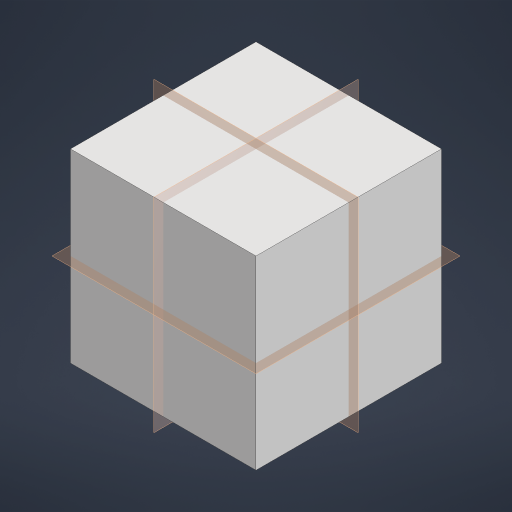
# Autodesk Inventor part: cube
Saved by Autodesk Inventor 2024 (Build 280153020, 153B)
## iProperties
Created: 2024-03-08
Part Number: cube
Material: Generic
Document SubType Name: Modeling
Designer: Oliver Read
Density: 1 g/cm^3
Appearance: Default
Author: Oliver Read
Autodesk Inventor part; units mm, degrees
(part 1 of 3)
sketch "Air Jet Form Tool" plane through (0, 0, 0) normal (0, 0, 1) x (1, 0, 0)
  line L0 (0.825, 4) -> (-0.795, 2.38)
  line L1 (-0.795, 2.38) -> (-2, 2.38)
  line L2 (-2, 2.38) -> (-2, 1.59)
  line L3 (-2, 1.59) -> (-4.8, 1.59)
  line L4 (-4.8, 1.59) -> (-4.8, 1.25)
  line L5 (-4.8, 1.25) -> (-8, 1.25)
  line L6 (-8, 1.25) -> (-9.25, 0)
  line L7 (0.825, 4) -> (0.825, 0)
  line L8 (0.825, 0) -> (-9.25, 0)
  point P0 (0, 0)
  point P1 (0, 0)
  point P2 (0, 3.175)
sketch "BS1 Centre Drill" plane through (0, 0, 0) normal (0, 0, 1) x (1, 0, 0)
  line L0 (0, 0) -> (1.5875, 0)
  line L1 (1.5875, 0) -> (0.595, -1.7191)
  line L2 (0.595, -1.7191) -> (0.595, -3.3455)
  line L3 (0.595, -3.3455) -> (0, -3.7031)
  line L4 (0, -3.7031) -> (0, 0)
sketch "BS2 Centre Drill" plane through (0, 0, 0) normal (0, 0, 1) x (1, 0, 0)
  line L0 (0, 0) -> (2.3812, 0)
  line L1 (2.3812, 0) -> (0.7937, -2.7496)
  line L2 (0.7937, -2.7496) -> (0.7938, -4.6349)
  line L3 (0.7938, -4.6349) -> (0, -5.1309)
  line L4 (0, -5.1309) -> (0, 0)
sketch "BS3 Centre Drill" plane through (0, 0, 0) normal (0, 0, 1) x (1, 0, 0)
  line L0 (0, 0) -> (3.175, 0)
  line L1 (3.175, 0) -> (1.1906, -3.437)
  line L2 (1.1906, -3.437) -> (1.1906, -6.6618)
  line L3 (1.1906, -6.6618) -> (0, -7.4058)
  line L4 (0, -7.4058) -> (0, 0)
sketch "BS4 Centre Drill" plane through (0, 0, 0) normal (0, 0, 1) x (1, 0, 0)
  line L0 (0, 0) -> (3.9688, 0)
  line L1 (3.9688, 0) -> (1.5875, -4.1244)
  line L2 (1.5875, -4.1244) -> (1.5875, -7.895)
  line L3 (1.5875, -7.895) -> (0, -8.8869)
  line L4 (0, -8.8869) -> (0, 0)
sketch "BS5 Centre Drill" plane through (0, 0, 0) normal (0, 0, 1) x (1, 0, 0)
  line L0 (0, 0) -> (5.5563, 0)
  line L1 (5.5563, 0) -> (2.3813, -5.4993)
  line L2 (2.3813, -5.4993) -> (2.3813, -11.155)
  line L3 (2.3813, -11.155) -> (0, -12.643)
  line L4 (0, -12.643) -> (0, 0)
sketch "CE - 5mm" plane through (0, 0, 0) normal (0, 0, 1) x (1, 0, 0)
  arc A0 (-0.75, 2.4875) -> (-0.75, -2.4875) centre (-1, 0) ccw
  arc A1 (-0.75, 1.7321) -> (-0.75, -1.7321) centre (-1, 0) ccw
  line L0 (-0.75, 1.7321) -> (-0.75, 2.4875)
  line L1 (-0.75, -2.4875) -> (-0.75, -1.7321)
  arc A2 (3.5, 2.4875) -> (3.5, -2.4875) centre (3.25, 0) ccw
  arc A3 (3.5, 1.7321) -> (1.5407, 0.375) centre (3.25, 0) ccw
  arc A4 (1.5407, -0.375) -> (3.5, -1.7321) centre (3.25, 0) ccw
  line L2 (3.5, 1.7321) -> (3.5, 2.4875)
  line L3 (3.5, -2.4875) -> (3.5, -1.7321)
  line L4 (3, -0.375) -> (3, 0.375)
  line L5 (1.5407, -0.375) -> (3, -0.375)
  line L6 (1.5407, 0.375) -> (3, 0.375)
  point P0 (0, 0)
sketch "UKCA - 5mm" plane through (0, 0, 0) normal (0, 0, 1) x (1, 0, 0)
  line L0 (1.0692, -0.2966) -> (0.6432, -0.2966) construction
  spline S0 degree 3 poles (1.0692, -0.2966) (0.6432, -0.2966) (0.2966, -0.6385) (0.2966, -1.0588) knots 1 1 1 1 2 2 2 2
  line L1 (0.6432, -0.2966) -> (0.2966, -0.6385) construction
  line L2 (0.2966, -0.6385) -> (0.2966, -1.0588) construction
  line L3 (0.2966, -1.0588) -> (0.2966, -2.5007)
  line L4 (0.2966, -2.5007) -> (0.7976, -2.5007)
  line L5 (-1.0692, 0.2966) -> (-1.7282, 0.2966)
  line L6 (0.7976, -1.9998) -> (1.9998, -1.9998)
  line L7 (1.9998, -1.9998) -> (1.9998, -2.5007)
  line L8 (1.9998, -2.5007) -> (2.5007, -2.5007)
  line L9 (2.5007, -2.5007) -> (2.5007, -1.0588)
  spline S1 degree 3 poles (2.5007, -1.0588) (2.5007, -0.6385) (2.1542, -0.2966) (1.7282, -0.2966) knots 9 9 9 9 10 10 10 10
  line L10 (2.5007, -1.0588) -> (2.5007, -0.6385) construction
  line L11 (2.5007, -0.6385) -> (2.1542, -0.2966) construction
  line L12 (2.1542, -0.2966) -> (1.7282, -0.2966) construction
  line L13 (0.7976, -2.5007) -> (0.7976, -1.9998)
  spline S2 degree 3 poles (0.7976, -1.0655) (0.7976, -0.9178) (0.9224, -0.7975) (1.0759, -0.7975) knots 1 1 1 1 2 2 2 2
  line L14 (0.7976, -1.0655) -> (0.7976, -0.9178) construction
  line L15 (0.7976, -0.9178) -> (0.9224, -0.7975) construction
  line L16 (0.9224, -0.7975) -> (1.0759, -0.7975) construction
  line L17 (1.0759, -0.7975) -> (1.7215, -0.7975)
  spline S3 degree 3 poles (1.7215, -0.7975) (1.8749, -0.7975) (1.9998, -0.9178) (1.9998, -1.0655) knots 3 3 3 3 4 4 4 4
  line L18 (1.7215, -0.7975) -> (1.8749, -0.7975) construction
  line L19 (1.8749, -0.7975) -> (1.9998, -0.9178) construction
  line L20 (1.9998, -0.9178) -> (1.9998, -1.0655) construction
  line L21 (1.9998, -1.0655) -> (1.9998, -1.4988)
  line L22 (1.9998, -1.4988) -> (0.7976, -1.4988)
  line L23 (0.7976, -1.4988) -> (0.7976, -1.0655)
  line L24 (-0.4795, 2.5007) -> (-0.4604, 2.5007)
  spline S4 degree 3 poles (-1.7282, 0.2966) (-2.1542, 0.2966) (-2.5007, 0.6386) (-2.5007, 1.0588) knots 1 1 1 1 2 2 2 2
  line L25 (-1.7282, 0.2966) -> (-2.1542, 0.2966) construction
  line L26 (-2.1542, 0.2966) -> (-2.5007, 0.6386) construction
  line L27 (-2.5007, 0.6386) -> (-2.5007, 1.0588) construction
  line L28 (-2.5007, 1.0588) -> (-2.5007, 2.5007)
  line L29 (-2.5007, 2.5007) -> (-1.9998, 2.5007)
  line L30 (-1.9998, 2.5007) -> (-1.9998, 1.0656)
  spline S5 degree 3 poles (-1.9998, 1.0656) (-1.9998, 0.9178) (-1.8749, 0.7976) (-1.7215, 0.7976) knots 5 5 5 5 6 6 6 6
  line L31 (-1.9998, 1.0656) -> (-1.9998, 0.9178) construction
  line L32 (-1.9998, 0.9178) -> (-1.8749, 0.7976) construction
  line L33 (-1.8749, 0.7976) -> (-1.7215, 0.7976) construction
  line L34 (-1.7215, 0.7976) -> (-1.0759, 0.7976)
  spline S6 degree 3 poles (-1.0759, 0.7976) (-0.9224, 0.7976) (-0.7976, 0.9178) (-0.7976, 1.0656) knots 7 7 7 7 8 8 8 8
  line L35 (-1.0759, 0.7976) -> (-0.9224, 0.7976) construction
  line L36 (-0.9224, 0.7976) -> (-0.7976, 0.9178) construction
  line L37 (-0.7976, 0.9178) -> (-0.7976, 1.0656) construction
  line L38 (-0.7976, 1.0656) -> (-0.7976, 2.5007)
  line L39 (-0.7976, 2.5007) -> (-0.2966, 2.5007)
  line L40 (-0.2966, 2.5007) -> (-0.2966, 1.0588)
  spline S7 degree 3 poles (-0.2966, 1.0588) (-0.2966, 0.6386) (-0.6432, 0.2966) (-1.0692, 0.2966) knots 11 11 11 11 12 12 12 12
  line L41 (-0.2966, 1.0588) -> (-0.2966, 0.6386) construction
  line L42 (-0.2966, 0.6386) -> (-0.6432, 0.2966) construction
  line L43 (-0.6432, 0.2966) -> (-1.0692, 0.2966) construction
  line L44 (2.5053, 2.5007) -> (1.8575, 2.5007)
  line L45 (1.8575, 2.5007) -> (0.7976, 1.6666)
  line L46 (0.7976, 1.6666) -> (0.7976, 2.5007)
  line L47 (0.7976, 2.5007) -> (0.2966, 2.5007)
  line L48 (0.2966, 2.5007) -> (0.2966, 0.2966)
  line L49 (0.2966, 0.2966) -> (0.7976, 0.2966)
  line L50 (0.7976, 0.2966) -> (0.7976, 1.1363)
  line L51 (0.7976, 1.1363) -> (1.8575, 0.2966)
  line L52 (1.8575, 0.2966) -> (2.5025, 0.2966)
  line L53 (2.5025, 0.2966) -> (1.1082, 1.4012)
  line L54 (1.1082, 1.4012) -> (2.5053, 2.5007)
  line L55 (-0.2966, -2.5007) -> (-1.7385, -2.5007)
  spline S8 degree 3 poles (-1.7385, -2.5007) (-2.1588, -2.5007) (-2.5007, -2.1474) (-2.5007, -1.7215) knots 1 1 1 1 2 2 2 2
  line L56 (-1.7385, -2.5007) -> (-2.1588, -2.5007) construction
  line L57 (-2.1588, -2.5007) -> (-2.5007, -2.1474) construction
  line L58 (-2.5007, -2.1474) -> (-2.5007, -1.7215) construction
  line L59 (-2.5007, -1.7215) -> (-2.5007, -1.0759)
  spline S9 degree 3 poles (-2.5007, -1.0759) (-2.5007, -0.6499) (-2.1588, -0.2966) (-1.7385, -0.2966) knots 3 3 3 3 4 4 4 4
  line L60 (-2.5007, -1.0759) -> (-2.5007, -0.6499) construction
  line L61 (-2.5007, -0.6499) -> (-2.1588, -0.2966) construction
  line L62 (-2.1588, -0.2966) -> (-1.7385, -0.2966) construction
  line L63 (-1.7385, -0.2966) -> (-0.2966, -0.2966)
  line L64 (-0.2966, -0.2966) -> (-0.2966, -0.7976)
  line L65 (-0.2966, -0.7976) -> (-1.7318, -0.7976)
  spline S10 degree 3 poles (-1.7318, -0.7976) (-1.8796, -0.7976) (-1.9998, -0.9224) (-1.9998, -1.0759) knots 7 7 7 7 8 8 8 8
  line L66 (-1.7318, -0.7976) -> (-1.8796, -0.7976) construction
  line L67 (-1.8796, -0.7976) -> (-1.9998, -0.9224) construction
  line L68 (-1.9998, -0.9224) -> (-1.9998, -1.0759) construction
  line L69 (-1.9998, -1.0759) -> (-1.9998, -1.7215)
  spline S11 degree 3 poles (-1.9998, -1.7215) (-1.9998, -1.8749) (-1.8796, -1.9998) (-1.7318, -1.9998) knots 9 9 9 9 10 10 10 10
  line L70 (-1.9998, -1.7215) -> (-1.9998, -1.8749) construction
  line L71 (-1.9998, -1.8749) -> (-1.8796, -1.9998) construction
  line L72 (-1.8796, -1.9998) -> (-1.7318, -1.9998) construction
  line L73 (-1.7318, -1.9998) -> (-0.2966, -1.9998)
  line L74 (-0.2966, -1.9998) -> (-0.2966, -2.5007)
  line L75 (1.7282, -0.2966) -> (1.0692, -0.2966)
  point P0 (0, 0)
sketch "WEEE - 5mm" plane through (0, 0, 0) normal (0, 0, 1) x (1, 0, 0)
  line L0 (1.7158, 2.5006) -> (1.7167, 2.5006)
  line L1 (-1.4262, -1.7883) -> (1.4264, -1.7883)
  line L2 (1.4264, -1.7883) -> (1.4264, -2.501)
  line L3 (1.4264, -2.501) -> (-1.4262, -2.501)
  circle A0 centre (0.5816, -0.4361) radius 0.0929
  arc A1 (0.5682, -0.1516) -> (0.3027, -0.4944) centre (0.5816, -0.4361) ccw
  arc A2 (0.3256, -0.5612) -> (0.8613, -0.382) centre (0.5816, -0.4361) ccw
  line L4 (0.3027, -0.4944) -> (-0.5023, -0.4944)
  line L5 (-0.5023, -0.4944) -> (-0.5485, 0.0433)
  line L6 (-0.5569, 0.1401) -> (-0.653, 1.2575)
  line L7 (-0.6619, 1.3613) -> (-0.6998, 1.8018)
  line L8 (0.3256, -0.5612) -> (-0.3706, -0.5612)
  line L9 (-0.3706, -0.5612) -> (-0.3706, -0.7192)
  line L10 (-0.3706, -0.7192) -> (-0.5415, -0.7192)
  line L11 (-0.5415, -0.7192) -> (-0.5415, -0.5602)
  arc A3 (-0.5811, -0.5036) -> (-0.5415, -0.5602) centre (-0.5214, -0.5041) ccw
  line L12 (-0.5811, -0.5041) -> (-0.6215, -0.0326)
  line L13 (-0.6299, 0.0642) -> (-0.7405, 1.3522)
  line L14 (-0.7494, 1.4557) -> (-0.7791, 1.8015)
  line L15 (-0.7791, 1.8015) -> (-0.9112, 1.8015)
  line L16 (-0.9112, 1.8015) -> (-0.9112, 1.8938)
  line L17 (-0.9112, 1.8938) -> (-0.7925, 1.8938)
  line L18 (-0.7139, 1.8938) -> (-0.6074, 1.8938)
  line L19 (-0.436, 1.8938) -> (0.7146, 1.8938)
  line L20 (-0.6998, 1.8018) -> (0.7133, 1.8018)
  line L21 (0.7133, 1.8018) -> (0.6996, 1.6165)
  line L22 (0.6751, 1.287) -> (0.5808, 0.0185)
  line L23 (0.5741, -0.0711) -> (0.5682, -0.1516)
  line L24 (0.7799, 1.8115) -> (0.7663, 1.6162)
  line L25 (0.7434, 1.287) -> (0.65, -0.0563)
  circle A4 centre (0.5816, -0.4361) radius 0.1555
  line L26 (-0.6074, 1.8938) -> (-0.6074, 2.0043)
  line L27 (-0.6074, 2.0851) -> (-0.6074, 2.1583)
  line L28 (-0.6074, 2.1583) -> (-0.436, 2.1583)
  line L29 (-0.436, 2.1583) -> (-0.436, 2.1445)
  line L30 (-0.436, 2.0657) -> (-0.436, 1.8938)
  arc A5 (-0.688, 1.9531) -> (-0.7139, 1.8938) centre (-0.6372, 1.8957) ccw
  arc A6 (-0.6074, 2.0043) -> (-0.688, 1.9531) centre (-0.3127, 1.4513) ccw
  arc A7 (-0.1585, 2.0919) -> (-0.436, 2.0657) centre (-0.1257, 0.2588) ccw
  arc A8 (-0.1585, 2.1706) -> (-0.436, 2.1445) centre (-0.1257, 0.3376) ccw
  line L31 (-0.1585, 2.2104) -> (-0.1585, 2.1706)
  line L32 (-0.1585, 2.0919) -> (-0.1585, 1.9995)
  line L33 (-0.1585, 1.9995) -> (0.2905, 1.9995)
  line L34 (0.2905, 1.9995) -> (0.2905, 2.0905)
  line L35 (0.2905, 2.1631) -> (0.2905, 2.2104)
  line L36 (0.2905, 2.2104) -> (-0.1585, 2.2104)
  line L37 (-0.0924, 2.1315) -> (-0.0924, 2.0789)
  line L38 (-0.0924, 2.0789) -> (0.2244, 2.0789)
  line L39 (0.2244, 2.0789) -> (0.2244, 2.1315)
  line L40 (0.2244, 2.1315) -> (-0.0924, 2.1315)
  arc A9 (-0.7663, 1.9743) -> (-0.7925, 1.8938) centre (-0.6917, 1.9054) ccw
  arc A10 (-0.6074, 2.0851) -> (-0.7663, 1.9743) centre (-0.2997, 1.4745) ccw
  arc A11 (0.7799, 1.8115) -> (0.7427, 1.9727) centre (0.8536, 1.9134) ccw
  arc A12 (0.6431, 1.9765) -> (0.4637, 2.0618) centre (0.3184, 1.5254) ccw
  arc A13 (0.7146, 1.8938) -> (0.6431, 1.9765) centre (0.5326, 1.8085) ccw
  arc A14 (0.617, 2.0738) -> (0.2905, 2.1631) centre (0.2581, 1.4034) ccw
  arc A15 (0.7427, 1.9727) -> (0.617, 2.0738) centre (0.3672, 1.6344) ccw
  arc A16 (0.4637, 2.0618) -> (0.2905, 2.0905) centre (0.1785, 0.8757) ccw
  line L41 (0.6603, 1.287) -> (0.6751, 1.287)
  line L42 (0.7434, 1.287) -> (0.9769, 1.287)
  line L43 (0.9769, 1.287) -> (0.9769, 1.6165)
  line L44 (0.6603, 1.6165) -> (0.6996, 1.6165)
  line L45 (0.7663, 1.6162) -> (0.8644, 1.6162)
  line L46 (0.9519, 1.6165) -> (0.9769, 1.6165)
  line L47 (0.6603, 1.6165) -> (0.6603, 1.4045)
  line L48 (0.6603, 1.3003) -> (0.6603, 1.287)
  line L49 (0.7522, 1.4058) -> (0.7522, 1.3659)
  line L50 (0.7522, 1.3659) -> (0.9112, 1.3659)
  line L51 (0.9112, 1.3659) -> (0.9112, 1.551)
  line L52 (0.9112, 1.551) -> (0.8981, 1.551)
  line L53 (0.7522, 1.4058) -> (0.8981, 1.551)
  line L54 (0.6603, 1.3003) -> (0.0153, 0.6296)
  line L55 (-1.4262, -2.501) -> (-1.4262, -1.7883)
  line L56 (-0.6215, -0.0326) -> (-1.6049, -1.0552)
  line L57 (-1.6049, -1.0552) -> (-1.657, -1.0028)
  line L58 (-1.657, -1.0028) -> (-0.6299, 0.0642)
  line L59 (-0.5569, 0.1401) -> (-0.0792, 0.6363)
  line L60 (-0.0342, 0.683) -> (0.3565, 1.0889)
  line L61 (0.4223, 1.1572) -> (0.6603, 1.4045)
  line L62 (0.8644, 1.6162) -> (1.7158, 2.5006)
  line L63 (1.7167, 2.5006) -> (1.7167, 2.4087)
  line L64 (1.7167, 2.4087) -> (0.9519, 1.6165)
  line L65 (0.4223, 1.1572) -> (0.4223, 1.2734)
  line L66 (0.4223, 1.2734) -> (-0.1717, 1.2734)
  line L67 (-0.0298, 0.5827) -> (-0.5485, 0.0433)
  line L68 (-0.1717, 1.0889) -> (0.3565, 1.0889)
  line L69 (-1.7167, 2.501) -> (-1.7167, 2.4092)
  line L70 (-1.7167, 2.4092) -> (-0.7405, 1.3522)
  line L71 (-0.653, 1.2575) -> (-0.0792, 0.6363)
  line L72 (-0.0298, 0.5827) -> (0.5741, -0.0711)
  line L73 (0.8613, -0.382) -> (1.4837, -1.0559)
  line L74 (1.4837, -1.0559) -> (1.533, -1.0104)
  line L75 (1.533, -1.0104) -> (0.65, -0.0563)
  line L76 (0.5808, 0.0185) -> (0.0153, 0.6296)
  line L77 (-0.0342, 0.683) -> (-0.6619, 1.3613)
  line L78 (-0.7494, 1.4557) -> (-1.7167, 2.501)
  line L79 (-0.1717, 1.2734) -> (-0.1717, 1.0889)
  point P0 (0, 0)
sketch "TELEC - 5mm" plane through (0, 0, 0) normal (0, 0, 1) x (1, 0, 0)
  arc A0 (0.4326, 0.6165) -> (0.3669, -0.8333) centre (-1.9901, 0) ccw
  arc A1 (0.0002, 0.8562) -> (-4.059, 0.6437) centre (-1.9901, 0) ccw
  line L0 (-3.3235, -0.8333) -> (-0.6568, -0.8333)
  line L1 (-0.6568, -0.8333) -> (-0.6568, -1.25)
  line L2 (-2.2401, -1.9167) -> (-1.7401, -1.9167)
  line L3 (-1.7401, -1.25) -> (-1.7401, -1.9167)
  line L4 (-1.7401, -1.25) -> (-0.6568, -1.25)
  line L5 (-2.2401, -1.25) -> (-2.2401, -1.9167)
  line L6 (-2.2401, -1.25) -> (-3.3235, -1.25)
  line L7 (-3.3235, -0.8333) -> (-3.3235, -1.25)
  line L8 (-3.3235, -0.5833) -> (-0.6568, -0.5833)
  line L9 (-0.6568, -0.5833) -> (-0.6568, -0.1667)
  line L10 (-3.3235, -0.5833) -> (-3.3235, -0.1667)
  line L11 (-3.3235, -0.1667) -> (-0.6568, -0.1667)
  line L12 (-2.1568, 0) -> (0.4326, 0.6165)
  line L13 (-4.1384, 0.2822) -> (-2.1568, 0.754)
  line L14 (-2.1568, 0) -> (-2.1568, 0.754)
  line L15 (-1.8235, 0.422) -> (0.0002, 0.8562)
  line L16 (-1.8235, 0.422) -> (-1.8235, 1.176)
  line L17 (-4.059, 0.6437) -> (-1.8235, 1.176)
  arc A2 (-4.1384, 0.2822) -> (0.0099, -0.8333) centre (-1.9901, 0) ccw
  line L18 (0.0099, -0.8333) -> (0.3669, -0.8333)
  line L19 (1.9123, 0.6959) -> (4.4042, 0.6959)
  line L20 (4.4042, 0.6959) -> (4.4042, -2.0609)
  line L21 (4.4042, -2.0609) -> (1.9123, -2.0609)
  line L22 (1.9123, -2.0609) -> (1.9123, 0.6959)
  line L23 (1.829, 0.7793) -> (4.4876, 0.7793)
  line L24 (4.4876, 0.7793) -> (4.4876, -2.1442)
  line L25 (4.4876, -2.1442) -> (1.829, -2.1442)
  line L26 (1.829, -2.1442) -> (1.829, 0.7793)
  line L27 (2.2996, 0.346) -> (2.2996, -1.7374)
  line L28 (2.2996, -1.7374) -> (2.7162, -1.7374)
  line L29 (2.7162, -1.7374) -> (2.7162, -0.8624)
  line L30 (2.7162, -0.8624) -> (2.9324, -0.8624)
  line L31 (3.6746, -1.7374) -> (4.1746, -1.7374)
  arc A3 (4.1746, -1.7374) -> (3.4751, -0.8264) centre (1.4812, -3.0813) ccw
  arc A4 (3.6746, -1.7374) -> (3.0775, -0.9212) centre (0.9812, -3.0813) ccw
  arc A5 (3.0775, -0.9212) -> (2.9324, -0.8624) centre (2.9324, -1.0707) ccw
  line L32 (2.7018, 0.015) -> (2.7018, -0.5017)
  arc A6 (3.3268, -0.5017) -> (3.3268, 0.015) centre (3.3268, -0.2433) ccw
  line L33 (2.7018, 0.015) -> (3.3268, 0.015)
  line L34 (3.3268, -0.5017) -> (2.7018, -0.5017)
  line L35 (2.2996, 0.346) -> (3.3895, 0.346)
  arc A7 (3.4751, -0.8264) -> (3.3895, 0.346) centre (3.3895, -0.2433) ccw
  point P0 (0, 0)
sketch "KCC - 5mm" plane through (0, 0, 0) normal (0, 0, 1) x (1, 0, 0)
  arc A0 (0.975, 0.9255) -> (0.975, -0.9255) centre (1.2235, 0) ccw
  arc A1 (1.0408, 0.9341) -> (0.975, 0.9255) centre (1.0408, 0.6805) ccw
  line L0 (1.0408, 0.9341) -> (1.6027, 0.9341)
  line L1 (1.6027, 0.9341) -> (1.6027, 0.6316)
  line L2 (1.6027, 0.6316) -> (1.1105, 0.6316)
  arc A2 (1.1105, 0.6316) -> (1.0378, 0.621) centre (1.1105, 0.378) ccw
  arc A3 (1.0378, 0.621) -> (1.0378, -0.621) centre (1.2235, 0) ccw
  arc A4 (1.0378, -0.621) -> (1.1105, -0.6316) centre (1.1105, -0.378) ccw
  line L3 (1.1105, -0.6316) -> (1.6027, -0.6316)
  line L4 (1.6027, -0.6316) -> (1.6027, -1.7334)
  line L5 (1.6027, -1.7334) -> (1.0569, -1.7334)
  arc A5 (1.0285, -1.7319) -> (1.0569, -1.7334) centre (1.0569, -1.4798) ccw
  arc A6 (1.0285, 1.7319) -> (1.0285, -1.7319) centre (1.2235, 0) ccw
  arc A7 (1.0569, 1.7334) -> (1.0285, 1.7319) centre (1.0569, 1.4798) ccw
  line L6 (1.0569, 1.7334) -> (1.2987, 1.7334)
  line L7 (1.2987, 1.7334) -> (1.2987, 2.179)
  line L8 (1.2987, 2.179) -> (1.0597, 2.179)
  arc A8 (1.0597, 2.179) -> (1.0382, 2.1781) centre (1.0597, 1.9253) ccw
  arc A9 (1.0382, 2.1781) -> (-0.8208, 0.774) centre (1.2235, 0) ccw
  line L9 (-0.8208, 0.774) -> (-0.8208, 2.1281)
  line L10 (-0.8208, 2.1281) -> (-1.2971, 2.1281)
  line L11 (-1.2971, 2.1281) -> (-1.2971, -2.1932)
  line L12 (-1.2971, -2.1932) -> (-0.8208, -2.1932)
  line L13 (-0.8208, -2.1932) -> (-0.8208, -0.774)
  arc A10 (-0.8208, -0.774) -> (1.0382, -2.1781) centre (1.2235, 0) ccw
  arc A11 (1.0382, -2.1781) -> (1.0597, -2.179) centre (1.0597, -1.9253) ccw
  line L14 (1.0597, -2.179) -> (1.6027, -2.179)
  line L15 (1.6027, -2.179) -> (1.6027, -2.5)
  line L16 (1.6027, -2.5) -> (0.9791, -2.5)
  arc A12 (0.9517, -2.4985) -> (0.9791, -2.5) centre (0.9791, -2.2463) ccw
  arc A13 (-0.5344, -1.7962) -> (0.9517, -2.4985) centre (1.2235, 0) ccw
  line L17 (-0.5344, -1.7962) -> (-0.5344, -2.5)
  line L18 (-0.5344, -2.5) -> (-1.6027, -2.5)
  line L19 (-1.6027, -2.5) -> (-1.6027, 2.5)
  line L20 (-1.6027, 2.5) -> (-0.5344, 2.5)
  line L21 (-0.5344, 2.5) -> (-0.5344, 1.7962)
  arc A14 (0.9517, 2.4985) -> (-0.5344, 1.7962) centre (1.2235, 0) ccw
  arc A15 (0.9791, 2.5) -> (0.9517, 2.4985) centre (0.9791, 2.2463) ccw
  line L22 (0.9791, 2.5) -> (1.6027, 2.5)
  line L23 (1.6027, 2.5) -> (1.6027, 1.4133)
  line L24 (1.6027, 1.4133) -> (1.0559, 1.4133)
  arc A16 (1.0559, 1.4133) -> (1.0196, 1.4107) centre (1.0559, 1.1596) ccw
  arc A17 (1.0196, 1.4107) -> (1.0196, -1.4107) centre (1.2235, 0) ccw
  arc A18 (1.0196, -1.4107) -> (1.0559, -1.4133) centre (1.0559, -1.1596) ccw
  line L25 (1.0559, -1.4133) -> (1.2987, -1.4133)
  line L26 (1.2987, -1.4133) -> (1.2987, -0.9341)
  line L27 (1.2987, -0.9341) -> (1.0408, -0.9341)
  arc A19 (0.975, -0.9255) -> (1.0408, -0.9341) centre (1.0408, -0.6805) ccw
  point P0 (0, 0)
sketch "Bowers Logo 1" plane through (0, 0, 0) normal (0, 0, 1) x (1, 0, 0)
  line L0 (0.7957, 3.45) -> (1.2479, 4.8418)
  line L1 (0.7957, 3.45) -> (1.2479, 4.8418)
  line L2 (-1.0969, 3.45) -> (0.7957, 3.45)
  line L3 (-1.0969, 3.45) -> (0.7957, 3.45)
  line L4 (-3.1926, -3) -> (-1.0969, 3.45)
  line L5 (-3.1926, -3) -> (-1.0969, 3.45)
  line L6 (-1.3, -3) -> (-3.1926, -3)
  line L7 (-1.3, -3) -> (-3.1926, -3)
  line L8 (-1.8363, -4.6506) -> (-1.3, -3)
  line L9 (-1.8363, -4.6506) -> (-1.3, -3)
  arc A0 (1.2479, 4.8418) -> (-1.8363, -4.6506) centre (0, 0) ccw
  line L10 (-1.8363, -4.6506) -> (-1.3, -3)
  line L11 (-1.3, -3) -> (-3.1926, -3)
  line L12 (-3.1926, -3) -> (-1.0969, 3.45)
  line L13 (-1.0969, 3.45) -> (0.7957, 3.45)
  line L14 (0.7957, 3.45) -> (1.2479, 4.8418)
  arc A1 (1.2479, 4.8418) -> (-1.8363, -4.6506) centre (0, 0) ccw
  line L15 (0.7957, 3.45) -> (1.2479, 4.8418)
  line L16 (-1.0969, 3.45) -> (0.7957, 3.45)
  line L17 (-3.1926, -3) -> (-1.0969, 3.45)
  line L18 (-1.3, -3) -> (-3.1926, -3)
  line L19 (-1.8363, -4.6506) -> (-1.3, -3)
  line L20 (2.1463, 4.5159) -> (1.8, 3.45)
  line L21 (2.1463, 4.5159) -> (1.8, 3.45)
  line L22 (-0.34, -3) -> (-0.9596, -4.907)
  line L23 (-0.34, -3) -> (-0.9596, -4.907)
  line L24 (1.76, -3) -> (-0.34, -3)
  line L25 (1.76, -3) -> (-0.34, -3)
  arc A2 (1.76, -3) -> (2.5364, 0.8349) centre (1.4, -0.9311) ccw
  line L26 (1.76, -3) -> (-0.34, -3)
  line L27 (-0.34, -3) -> (-0.9596, -4.907)
  arc A3 (-0.9596, -4.907) -> (2.1463, 4.5159) centre (0, 0) ccw
  line L28 (2.1463, 4.5159) -> (1.8, 3.45)
  arc A4 (2.5364, 0.8349) -> (1.8, 3.45) centre (1.5559, 1.97) ccw
  arc A5 (1.76, -3) -> (2.5364, 0.8349) centre (1.4, -0.9311) ccw
  arc A6 (2.5364, 0.8349) -> (1.8, 3.45) centre (1.5559, 1.97) ccw
  line L29 (2.1463, 4.5159) -> (1.8, 3.45)
  arc A7 (-0.9596, -4.907) -> (2.1463, 4.5159) centre (0, 0) ccw
  line L30 (-0.34, -3) -> (-0.9596, -4.907)
  line L31 (1.76, -3) -> (-0.34, -3)
  line L32 (-0.34, -3) -> (1.8, 3.45)
  line L33 (-0.34, -3) -> (1.8, 3.45)
  line L34 (-1.3, -3) -> (-0.34, -3)
  line L35 (-1.3, -3) -> (-0.34, -3)
  line L36 (0.7957, 3.45) -> (-1.3, -3)
  line L37 (0.7957, 3.45) -> (-1.3, -3)
  line L38 (1.8, 3.45) -> (0.7957, 3.45)
  line L39 (1.8, 3.45) -> (0.7957, 3.45)
  line L40 (1.8, 3.45) -> (0.7957, 3.45)
  line L41 (0.7957, 3.45) -> (-1.3, -3)
  line L42 (-1.3, -3) -> (-0.34, -3)
  line L43 (-0.34, -3) -> (1.8, 3.45)
  line L44 (1.8, 3.45) -> (0.7957, 3.45)
  line L45 (-0.34, -3) -> (1.8, 3.45)
  line L46 (-1.3, -3) -> (-0.34, -3)
  line L47 (0.7957, 3.45) -> (-1.3, -3)
  point P0 (0, 0)
sketch "Bowers Logo 2" plane through (0, 0, 0) normal (0, 0, 1) x (1, 0, 0)
  arc A0 (-15.0251, -2.8294) -> (-14.9267, -1.9003) centre (-15.0392, -2.3581) ccw
  line L0 (-15.0251, -2.8294) -> (-15.6547, -2.8294)
  line L1 (-14.9267, -1.9003) -> (-15.4912, -1.9003)
  line L2 (10.3315, -2.1386) -> (10.4158, -2.1472)
  line L3 (10.4158, -2.1472) -> (10.3315, -2.1386)
  line L4 (10.4158, -2.1472) -> (10.4958, -2.1638)
  line L5 (10.4958, -2.1638) -> (10.4158, -2.1472)
  line L6 (10.4958, -2.1638) -> (10.573, -2.189)
  line L7 (10.573, -2.189) -> (10.4958, -2.1638)
  line L8 (10.573, -2.189) -> (10.6458, -2.2222)
  line L9 (10.6458, -2.2222) -> (10.573, -2.189)
  line L10 (10.6458, -2.2222) -> (10.715, -2.2647)
  line L11 (10.715, -2.2647) -> (10.6458, -2.2222)
  line L12 (10.715, -2.2647) -> (10.7806, -2.3152)
  line L13 (10.7806, -2.3152) -> (10.715, -2.2647)
  line L14 (10.7806, -2.3152) -> (10.8419, -2.3743)
  line L15 (10.8419, -2.3743) -> (10.7806, -2.3152)
  line L16 (10.8419, -2.3743) -> (10.8578, -2.3909)
  line L17 (10.8578, -2.3909) -> (10.8419, -2.3743)
  line L18 (10.8578, -2.3909) -> (10.9061, -2.4522)
  line L19 (10.9061, -2.4522) -> (10.8578, -2.3909)
  line L20 (10.9061, -2.4522) -> (10.9479, -2.5178)
  line L21 (10.9479, -2.5178) -> (10.9061, -2.4522)
  line L22 (10.9479, -2.5178) -> (10.9832, -2.5877)
  line L23 (10.9832, -2.5877) -> (10.9479, -2.5178)
  line L24 (10.9832, -2.5877) -> (11.0128, -2.6627)
  line L25 (11.0128, -2.6627) -> (10.9832, -2.5877)
  line L26 (11.0128, -2.6627) -> (11.0351, -2.742)
  line L27 (11.0351, -2.742) -> (11.0128, -2.6627)
  line L28 (11.0351, -2.742) -> (11.051, -2.8264)
  line L29 (11.051, -2.8264) -> (11.0351, -2.742)
  line L30 (11.051, -2.8264) -> (11.0611, -2.9151)
  line L31 (11.0611, -2.9151) -> (11.051, -2.8264)
  line L32 (11.0611, -2.9151) -> (11.064, -3.0088)
  line L33 (11.064, -3.0088) -> (11.0611, -2.9151)
  line L34 (11.064, -3.0088) -> (11.0618, -3.0902)
  line L35 (11.0618, -3.0902) -> (11.064, -3.0088)
  line L36 (11.0618, -3.0902) -> (11.0546, -3.1732)
  line L37 (11.0546, -3.1732) -> (11.0618, -3.0902)
  line L38 (11.0546, -3.1732) -> (11.0431, -3.2561)
  line L39 (11.0431, -3.2561) -> (11.0546, -3.1732)
  line L40 (11.0431, -3.2561) -> (11.0272, -3.3397)
  line L41 (11.0272, -3.3397) -> (11.0431, -3.2561)
  line L42 (11.0272, -3.3397) -> (11.0063, -3.4233)
  line L43 (11.0063, -3.4233) -> (11.0272, -3.3397)
  line L44 (11.0063, -3.4233) -> (10.9803, -3.5077)
  line L45 (10.9803, -3.5077) -> (11.0063, -3.4233)
  line L46 (10.9803, -3.5077) -> (10.9565, -3.5747)
  line L47 (10.9565, -3.5747) -> (10.9803, -3.5077)
  line L48 (10.9565, -3.5747) -> (10.9219, -3.6562)
  line L49 (10.9219, -3.6562) -> (10.9565, -3.5747)
  line L50 (10.9219, -3.6562) -> (10.8844, -3.7333)
  line L51 (10.8844, -3.7333) -> (10.9219, -3.6562)
  line L52 (10.8844, -3.7333) -> (10.8433, -3.8054)
  line L53 (10.8433, -3.8054) -> (10.8844, -3.7333)
  line L54 (10.8433, -3.8054) -> (10.7979, -3.8725)
  line L55 (10.7979, -3.8725) -> (10.8433, -3.8054)
  line L56 (10.7979, -3.8725) -> (10.7496, -3.9352)
  line L57 (10.7496, -3.9352) -> (10.7979, -3.8725)
  line L58 (10.7496, -3.9352) -> (10.7431, -3.9424)
  line L59 (10.7431, -3.9424) -> (10.7496, -3.9352)
  line L60 (10.7431, -3.9424) -> (10.684, -4.0073)
  line L61 (10.684, -4.0073) -> (10.7431, -3.9424)
  line L62 (10.684, -4.0073) -> (10.6213, -4.0657)
  line L63 (10.6213, -4.0657) -> (10.684, -4.0073)
  line L64 (10.6213, -4.0657) -> (10.5564, -4.1183)
  line L65 (10.5564, -4.1183) -> (10.6213, -4.0657)
  line L66 (10.5564, -4.1183) -> (10.4879, -4.1652)
  line L67 (10.4879, -4.1652) -> (10.5564, -4.1183)
  line L68 (10.4879, -4.1652) -> (10.4165, -4.2063)
  line L69 (10.4165, -4.2063) -> (10.4879, -4.1652)
  line L70 (10.4165, -4.2063) -> (10.3524, -4.2366)
  line L71 (10.3524, -4.2366) -> (10.4165, -4.2063)
  line L72 (10.3524, -4.2366) -> (10.2731, -4.2661)
  line L73 (10.2731, -4.2661) -> (10.3524, -4.2366)
  line L74 (10.2731, -4.2661) -> (10.1923, -4.287)
  line L75 (10.1923, -4.287) -> (10.2731, -4.2661)
  line L76 (10.1923, -4.287) -> (10.1101, -4.3)
  line L77 (10.1101, -4.3) -> (10.1923, -4.287)
  line L78 (10.1101, -4.3) -> (10.0258, -4.3043)
  line L79 (10.0258, -4.3043) -> (10.1101, -4.3)
  line L80 (10.0258, -4.3043) -> (10.0215, -4.3043)
  line L81 (10.0215, -4.3043) -> (10.0258, -4.3043)
  line L82 (10.0215, -4.3043) -> (9.9378, -4.2993)
  line L83 (9.9378, -4.2993) -> (10.0215, -4.3043)
  line L84 (9.9378, -4.2993) -> (9.8564, -4.2856)
  line L85 (9.8564, -4.2856) -> (9.9378, -4.2993)
  line L86 (9.8564, -4.2856) -> (9.7763, -4.264)
  line L87 (9.7763, -4.264) -> (9.8564, -4.2856)
  line L88 (9.7763, -4.264) -> (9.6978, -4.233)
  line L89 (9.6978, -4.233) -> (9.7763, -4.264)
  line L90 (9.6978, -4.233) -> (9.6206, -4.1933)
  line L91 (9.6206, -4.1933) -> (9.6978, -4.233)
  line L92 (9.6206, -4.1933) -> (9.6127, -4.1883)
  line L93 (9.6127, -4.1883) -> (9.6206, -4.1933)
  line L94 (9.6127, -4.1883) -> (9.5413, -4.1407)
  line L95 (9.5413, -4.1407) -> (9.6127, -4.1883)
  line L96 (9.5413, -4.1407) -> (9.4779, -4.0873)
  line L97 (9.4779, -4.0873) -> (9.5413, -4.1407)
  line L98 (9.4779, -4.0873) -> (9.4216, -4.0268)
  line L99 (9.4216, -4.0268) -> (9.4779, -4.0873)
  line L100 (9.4216, -4.0268) -> (9.3726, -3.9597)
  line L101 (9.3726, -3.9597) -> (9.4216, -4.0268)
  line L102 (9.3726, -3.9597) -> (9.3315, -3.8855)
  line L103 (9.3315, -3.8855) -> (9.3726, -3.9597)
  line L104 (9.3315, -3.8855) -> (9.3214, -3.8638)
  line L105 (9.3214, -3.8638) -> (9.3315, -3.8855)
  line L106 (9.3214, -3.8638) -> (9.2897, -3.7874)
  line L107 (9.2897, -3.7874) -> (9.3214, -3.8638)
  line L108 (9.2897, -3.7874) -> (9.2652, -3.7088)
  line L109 (9.2652, -3.7088) -> (9.2897, -3.7874)
  line L110 (9.2652, -3.7088) -> (9.2472, -3.6266)
  line L111 (9.2472, -3.6266) -> (9.2652, -3.7088)
  line L112 (9.2472, -3.6266) -> (9.2371, -3.5423)
  line L113 (9.2371, -3.5423) -> (9.2472, -3.6266)
  line L114 (9.2371, -3.5423) -> (9.2335, -3.455)
  line L115 (9.2335, -3.455) -> (9.2371, -3.5423)
  line L116 (9.2335, -3.455) -> (9.2335, -3.4118)
  line L117 (9.2335, -3.4118) -> (9.2335, -3.455)
  line L118 (9.2335, -3.4118) -> (9.2378, -3.3181)
  line L119 (9.2378, -3.3181) -> (9.2335, -3.4118)
  line L120 (9.2378, -3.3181) -> (9.2457, -3.2279)
  line L121 (9.2457, -3.2279) -> (9.2378, -3.3181)
  line L122 (9.2457, -3.2279) -> (9.258, -3.14)
  line L123 (9.258, -3.14) -> (9.2457, -3.2279)
  line L124 (9.258, -3.14) -> (9.2738, -3.0556)
  line L125 (9.2738, -3.0556) -> (9.258, -3.14)
  line L126 (9.2738, -3.0556) -> (9.2947, -2.9749)
  line L127 (9.2947, -2.9749) -> (9.2738, -3.0556)
  line L128 (9.2947, -2.9749) -> (9.3192, -2.8963)
  line L129 (9.3192, -2.8963) -> (9.2947, -2.9749)
  line L130 (9.3192, -2.8963) -> (9.3481, -2.8213)
  line L131 (9.3481, -2.8213) -> (9.3192, -2.8963)
  line L132 (9.3481, -2.8213) -> (9.3805, -2.75)
  line L133 (9.3805, -2.75) -> (9.3481, -2.8213)
  line L134 (9.3805, -2.75) -> (9.4173, -2.6815)
  line L135 (9.4173, -2.6815) -> (9.3805, -2.75)
  line L136 (9.4173, -2.6815) -> (9.4584, -2.6159)
  line L137 (9.4584, -2.6159) -> (9.4173, -2.6815)
  line L138 (9.4584, -2.6159) -> (9.5038, -2.5539)
  line L139 (9.5038, -2.5539) -> (9.4584, -2.6159)
  line L140 (9.5038, -2.5539) -> (9.5536, -2.494)
  line L141 (9.5536, -2.494) -> (9.5038, -2.5539)
  line L142 (9.5536, -2.494) -> (9.5687, -2.4774)
  line L143 (9.5687, -2.4774) -> (9.5536, -2.494)
  line L144 (9.5687, -2.4774) -> (9.6321, -2.4133)
  line L145 (9.6321, -2.4133) -> (9.5687, -2.4774)
  line L146 (9.6321, -2.4133) -> (9.6978, -2.3556)
  line L147 (9.6978, -2.3556) -> (9.6321, -2.4133)
  line L148 (9.6978, -2.3556) -> (9.7655, -2.3044)
  line L149 (9.7655, -2.3044) -> (9.6978, -2.3556)
  line L150 (9.7655, -2.3044) -> (9.8355, -2.2604)
  line L151 (9.8355, -2.2604) -> (9.7655, -2.3044)
  line L152 (9.8355, -2.2604) -> (9.9068, -2.2229)
  line L153 (9.9068, -2.2229) -> (9.8355, -2.2604)
  line L154 (9.9068, -2.2229) -> (9.9796, -2.1919)
  line L155 (9.9796, -2.1919) -> (9.9068, -2.2229)
  line L156 (9.9796, -2.1919) -> (10.0546, -2.1681)
  line L157 (10.0546, -2.1681) -> (9.9796, -2.1919)
  line L158 (10.0546, -2.1681) -> (10.1318, -2.1516)
  line L159 (10.1318, -2.1516) -> (10.0546, -2.1681)
  line L160 (10.1318, -2.1516) -> (10.2104, -2.1415)
  line L161 (10.2104, -2.1415) -> (10.1318, -2.1516)
  line L162 (10.2104, -2.1415) -> (10.2911, -2.1379)
  line L163 (10.2911, -2.1379) -> (10.2104, -2.1415)
  line L164 (10.2911, -2.1379) -> (10.3315, -2.1386)
  line L165 (10.3315, -2.1386) -> (10.2911, -2.1379)
  line L166 (10.2911, -2.1379) -> (10.3315, -2.1386)
  line L167 (10.3315, -2.1386) -> (10.4158, -2.1472)
  line L168 (10.4158, -2.1472) -> (10.4958, -2.1638)
  line L169 (10.4958, -2.1638) -> (10.573, -2.189)
  line L170 (10.573, -2.189) -> (10.6458, -2.2222)
  line L171 (10.6458, -2.2222) -> (10.715, -2.2647)
  line L172 (10.715, -2.2647) -> (10.7806, -2.3152)
  line L173 (10.7806, -2.3152) -> (10.8419, -2.3743)
  line L174 (10.8419, -2.3743) -> (10.8578, -2.3909)
  line L175 (10.8578, -2.3909) -> (10.9061, -2.4522)
  line L176 (10.9061, -2.4522) -> (10.9479, -2.5178)
  line L177 (10.9479, -2.5178) -> (10.9832, -2.5877)
  line L178 (10.9832, -2.5877) -> (11.0128, -2.6627)
  line L179 (11.0128, -2.6627) -> (11.0351, -2.742)
  line L180 (11.0351, -2.742) -> (11.051, -2.8264)
  line L181 (11.051, -2.8264) -> (11.0611, -2.9151)
  line L182 (11.0611, -2.9151) -> (11.064, -3.0088)
  line L183 (11.064, -3.0088) -> (11.0618, -3.0902)
  line L184 (11.0618, -3.0902) -> (11.0546, -3.1732)
  line L185 (11.0546, -3.1732) -> (11.0431, -3.2561)
  line L186 (11.0431, -3.2561) -> (11.0272, -3.3397)
  line L187 (11.0272, -3.3397) -> (11.0063, -3.4233)
  line L188 (11.0063, -3.4233) -> (10.9803, -3.5077)
  line L189 (10.9803, -3.5077) -> (10.9565, -3.5747)
  line L190 (10.9565, -3.5747) -> (10.9219, -3.6562)
  line L191 (10.9219, -3.6562) -> (10.8844, -3.7333)
  line L192 (10.8844, -3.7333) -> (10.8433, -3.8054)
  line L193 (10.8433, -3.8054) -> (10.7979, -3.8725)
  line L194 (10.7979, -3.8725) -> (10.7496, -3.9352)
  line L195 (10.7496, -3.9352) -> (10.7431, -3.9424)
  line L196 (10.7431, -3.9424) -> (10.684, -4.0073)
  line L197 (10.684, -4.0073) -> (10.6213, -4.0657)
  line L198 (10.6213, -4.0657) -> (10.5564, -4.1183)
  line L199 (10.5564, -4.1183) -> (10.4879, -4.1652)
  line L200 (10.4879, -4.1652) -> (10.4165, -4.2063)
  line L201 (10.4165, -4.2063) -> (10.3524, -4.2366)
  line L202 (10.3524, -4.2366) -> (10.2731, -4.2661)
  line L203 (10.2731, -4.2661) -> (10.1923, -4.287)
  line L204 (10.1923, -4.287) -> (10.1101, -4.3)
  line L205 (10.1101, -4.3) -> (10.0258, -4.3043)
  line L206 (10.0258, -4.3043) -> (10.0215, -4.3043)
  line L207 (10.0215, -4.3043) -> (9.9378, -4.2993)
  line L208 (9.9378, -4.2993) -> (9.8564, -4.2856)
  line L209 (9.8564, -4.2856) -> (9.7763, -4.264)
  line L210 (9.7763, -4.264) -> (9.6978, -4.233)
  line L211 (9.6978, -4.233) -> (9.6206, -4.1933)
  line L212 (9.6206, -4.1933) -> (9.6127, -4.1883)
  line L213 (9.6127, -4.1883) -> (9.5413, -4.1407)
  line L214 (9.5413, -4.1407) -> (9.4779, -4.0873)
  line L215 (9.4779, -4.0873) -> (9.4216, -4.0268)
  line L216 (9.4216, -4.0268) -> (9.3726, -3.9597)
  line L217 (9.3726, -3.9597) -> (9.3315, -3.8855)
  line L218 (9.3315, -3.8855) -> (9.3214, -3.8638)
  line L219 (9.3214, -3.8638) -> (9.2897, -3.7874)
  line L220 (9.2897, -3.7874) -> (9.2652, -3.7088)
  line L221 (9.2652, -3.7088) -> (9.2472, -3.6266)
  line L222 (9.2472, -3.6266) -> (9.2371, -3.5423)
  line L223 (9.2371, -3.5423) -> (9.2335, -3.455)
  line L224 (9.2335, -3.455) -> (9.2335, -3.4118)
  line L225 (9.2335, -3.4118) -> (9.2378, -3.3181)
  line L226 (9.2378, -3.3181) -> (9.2457, -3.2279)
  line L227 (9.2457, -3.2279) -> (9.258, -3.14)
  line L228 (9.258, -3.14) -> (9.2738, -3.0556)
  line L229 (9.2738, -3.0556) -> (9.2947, -2.9749)
  line L230 (9.2947, -2.9749) -> (9.3192, -2.8963)
  line L231 (9.3192, -2.8963) -> (9.3481, -2.8213)
  line L232 (9.3481, -2.8213) -> (9.3805, -2.75)
  line L233 (9.3805, -2.75) -> (9.4173, -2.6815)
  line L234 (9.4173, -2.6815) -> (9.4584, -2.6159)
  line L235 (9.4584, -2.6159) -> (9.5038, -2.5539)
  line L236 (9.5038, -2.5539) -> (9.5536, -2.494)
  line L237 (9.5536, -2.494) -> (9.5687, -2.4774)
  line L238 (9.5687, -2.4774) -> (9.6321, -2.4133)
  line L239 (9.6321, -2.4133) -> (9.6978, -2.3556)
  line L240 (9.6978, -2.3556) -> (9.7655, -2.3044)
  line L241 (9.7655, -2.3044) -> (9.8355, -2.2604)
  line L242 (9.8355, -2.2604) -> (9.9068, -2.2229)
  line L243 (9.9068, -2.2229) -> (9.9796, -2.1919)
  line L244 (9.9796, -2.1919) -> (10.0546, -2.1681)
  line L245 (10.0546, -2.1681) -> (10.1318, -2.1516)
  line L246 (10.1318, -2.1516) -> (10.2104, -2.1415)
  line L247 (10.2104, -2.1415) -> (10.2911, -2.1379)
  line L248 (10.3315, -2.1386) -> (10.2911, -2.1379)
  line L249 (10.2911, -2.1379) -> (10.2104, -2.1415)
  line L250 (10.2104, -2.1415) -> (10.1318, -2.1516)
  line L251 (10.1318, -2.1516) -> (10.0546, -2.1681)
  line L252 (10.0546, -2.1681) -> (9.9796, -2.1919)
  line L253 (9.9796, -2.1919) -> (9.9068, -2.2229)
  line L254 (9.9068, -2.2229) -> (9.8355, -2.2604)
  line L255 (9.8355, -2.2604) -> (9.7655, -2.3044)
  line L256 (9.7655, -2.3044) -> (9.6978, -2.3556)
  line L257 (9.6978, -2.3556) -> (9.6321, -2.4133)
  line L258 (9.6321, -2.4133) -> (9.5687, -2.4774)
  line L259 (9.5687, -2.4774) -> (9.5536, -2.494)
  line L260 (9.5536, -2.494) -> (9.5038, -2.5539)
  line L261 (9.5038, -2.5539) -> (9.4584, -2.6159)
  line L262 (9.4584, -2.6159) -> (9.4173, -2.6815)
  line L263 (9.4173, -2.6815) -> (9.3805, -2.75)
  line L264 (9.3805, -2.75) -> (9.3481, -2.8213)
  line L265 (9.3481, -2.8213) -> (9.3192, -2.8963)
  line L266 (9.3192, -2.8963) -> (9.2947, -2.9749)
  line L267 (9.2947, -2.9749) -> (9.2738, -3.0556)
  line L268 (9.2738, -3.0556) -> (9.258, -3.14)
  line L269 (9.258, -3.14) -> (9.2457, -3.2279)
  line L270 (9.2457, -3.2279) -> (9.2378, -3.3181)
  line L271 (9.2378, -3.3181) -> (9.2335, -3.4118)
  line L272 (9.2335, -3.4118) -> (9.2335, -3.455)
  line L273 (9.2335, -3.455) -> (9.2371, -3.5423)
  line L274 (9.2371, -3.5423) -> (9.2472, -3.6266)
  line L275 (9.2472, -3.6266) -> (9.2652, -3.7088)
  line L276 (9.2652, -3.7088) -> (9.2897, -3.7874)
  line L277 (9.2897, -3.7874) -> (9.3214, -3.8638)
  line L278 (9.3214, -3.8638) -> (9.3315, -3.8855)
  line L279 (9.3315, -3.8855) -> (9.3726, -3.9597)
  line L280 (9.3726, -3.9597) -> (9.4216, -4.0268)
  line L281 (9.4216, -4.0268) -> (9.4779, -4.0873)
  line L282 (9.4779, -4.0873) -> (9.5413, -4.1407)
  line L283 (9.5413, -4.1407) -> (9.6127, -4.1883)
  line L284 (9.6127, -4.1883) -> (9.6206, -4.1933)
  line L285 (9.6206, -4.1933) -> (9.6978, -4.233)
  line L286 (9.6978, -4.233) -> (9.7763, -4.264)
  line L287 (9.7763, -4.264) -> (9.8564, -4.2856)
  line L288 (9.8564, -4.2856) -> (9.9378, -4.2993)
  line L289 (9.9378, -4.2993) -> (10.0215, -4.3043)
  line L290 (10.0215, -4.3043) -> (10.0258, -4.3043)
  line L291 (10.0258, -4.3043) -> (10.1101, -4.3)
  line L292 (10.1101, -4.3) -> (10.1923, -4.287)
  line L293 (10.1923, -4.287) -> (10.2731, -4.2661)
  line L294 (10.2731, -4.2661) -> (10.3524, -4.2366)
  line L295 (10.3524, -4.2366) -> (10.4165, -4.2063)
  line L296 (10.4165, -4.2063) -> (10.4879, -4.1652)
  line L297 (10.4879, -4.1652) -> (10.5564, -4.1183)
  line L298 (10.5564, -4.1183) -> (10.6213, -4.0657)
  line L299 (10.6213, -4.0657) -> (10.684, -4.0073)
  line L300 (10.684, -4.0073) -> (10.7431, -3.9424)
  line L301 (10.7431, -3.9424) -> (10.7496, -3.9352)
  line L302 (10.7496, -3.9352) -> (10.7979, -3.8725)
  line L303 (10.7979, -3.8725) -> (10.8433, -3.8054)
  line L304 (10.8433, -3.8054) -> (10.8844, -3.7333)
  line L305 (10.8844, -3.7333) -> (10.9219, -3.6562)
  line L306 (10.9219, -3.6562) -> (10.9565, -3.5747)
  line L307 (10.9565, -3.5747) -> (10.9803, -3.5077)
  line L308 (10.9803, -3.5077) -> (11.0063, -3.4233)
  line L309 (11.0063, -3.4233) -> (11.0272, -3.3397)
  line L310 (11.0272, -3.3397) -> (11.0431, -3.2561)
  line L311 (11.0431, -3.2561) -> (11.0546, -3.1732)
  line L312 (11.0546, -3.1732) -> (11.0618, -3.0902)
  line L313 (11.0618, -3.0902) -> (11.064, -3.0088)
  line L314 (11.064, -3.0088) -> (11.0611, -2.9151)
  line L315 (11.0611, -2.9151) -> (11.051, -2.8264)
  line L316 (11.051, -2.8264) -> (11.0351, -2.742)
  line L317 (11.0351, -2.742) -> (11.0128, -2.6627)
  line L318 (11.0128, -2.6627) -> (10.9832, -2.5877)
  line L319 (10.9832, -2.5877) -> (10.9479, -2.5178)
  line L320 (10.9479, -2.5178) -> (10.9061, -2.4522)
  line L321 (10.9061, -2.4522) -> (10.8578, -2.3909)
  line L322 (10.8578, -2.3909) -> (10.8419, -2.3743)
  line L323 (10.8419, -2.3743) -> (10.7806, -2.3152)
  line L324 (10.7806, -2.3152) -> (10.715, -2.2647)
  line L325 (10.715, -2.2647) -> (10.6458, -2.2222)
  line L326 (10.6458, -2.2222) -> (10.573, -2.189)
  line L327 (10.573, -2.189) -> (10.4958, -2.1638)
  line L328 (10.4958, -2.1638) -> (10.4158, -2.1472)
  line L329 (10.4158, -2.1472) -> (10.3315, -2.1386)
  line L330 (7.8031, -2.1804) -> (7.9026, -2.1854)
  line L331 (7.9026, -2.1854) -> (7.8031, -2.1804)
  line L332 (7.9026, -2.1854) -> (7.9819, -2.1955)
  line L333 (7.9819, -2.1955) -> (7.9026, -2.1854)
  line L334 (7.9819, -2.1955) -> (8.041, -2.2107)
  line L335 (8.041, -2.2107) -> (7.9819, -2.1955)
  line L336 (8.041, -2.2107) -> (8.0561, -2.2172)
  line L337 (8.0561, -2.2172) -> (8.041, -2.2107)
  line L338 (8.0561, -2.2172) -> (8.1246, -2.2604)
  line L339 (8.1246, -2.2604) -> (8.0561, -2.2172)
  line L340 (8.1246, -2.2604) -> (8.1787, -2.3268)
  line L341 (8.1787, -2.3268) -> (8.1246, -2.2604)
  line L342 (8.1787, -2.3268) -> (8.1989, -2.365)
  line L343 (8.1989, -2.365) -> (8.1787, -2.3268)
  line L344 (8.1989, -2.365) -> (8.2234, -2.4435)
  line L345 (8.2234, -2.4435) -> (8.1989, -2.365)
  line L346 (8.2234, -2.4435) -> (8.2313, -2.5308)
  line L347 (8.2313, -2.5308) -> (8.2234, -2.4435)
  line L348 (8.2313, -2.5308) -> (8.2313, -2.5495)
  line L349 (8.2313, -2.5495) -> (8.2313, -2.5308)
  line L350 (8.2313, -2.5495) -> (8.2212, -2.6332)
  line L351 (8.2212, -2.6332) -> (8.2313, -2.5495)
  line L352 (8.2212, -2.6332) -> (8.1982, -2.7125)
  line L353 (8.1982, -2.7125) -> (8.2212, -2.6332)
  line L354 (8.1982, -2.7125) -> (8.1607, -2.7889)
  line L355 (8.1607, -2.7889) -> (8.1982, -2.7125)
  line L356 (8.1607, -2.7889) -> (8.1463, -2.812)
  line L357 (8.1463, -2.812) -> (8.1607, -2.7889)
  line L358 (8.1463, -2.812) -> (8.0951, -2.8768)
  line L359 (8.0951, -2.8768) -> (8.1463, -2.812)
  line L360 (8.0951, -2.8768) -> (8.0331, -2.9331)
  line L361 (8.0331, -2.9331) -> (8.0951, -2.8768)
  line L362 (8.0331, -2.9331) -> (7.961, -2.9799)
  line L363 (7.961, -2.9799) -> (8.0331, -2.9331)
  line L364 (7.961, -2.9799) -> (7.9552, -2.9828)
  line L365 (7.9552, -2.9828) -> (7.961, -2.9799)
  line L366 (7.9552, -2.9828) -> (7.8867, -3.0138)
  line L367 (7.8867, -3.0138) -> (7.9552, -2.9828)
  line L368 (7.8867, -3.0138) -> (7.8103, -3.0391)
  line L369 (7.8103, -3.0391) -> (7.8867, -3.0138)
  line L370 (7.8103, -3.0391) -> (7.7245, -3.0578)
  line L371 (7.7245, -3.0578) -> (7.8103, -3.0391)
  line L372 (7.7245, -3.0578) -> (7.6301, -3.0708)
  line L373 (7.6301, -3.0708) -> (7.7245, -3.0578)
  line L374 (7.6301, -3.0708) -> (7.62, -3.0715)
  line L375 (7.62, -3.0715) -> (7.6301, -3.0708)
  line L376 (7.62, -3.0715) -> (7.5673, -3.0744)
  line L377 (7.5673, -3.0744) -> (7.62, -3.0715)
  line L378 (7.5673, -3.0744) -> (7.4981, -3.0773)
  line L379 (7.4981, -3.0773) -> (7.5673, -3.0744)
  line L380 (7.4981, -3.0773) -> (7.4109, -3.0787)
  line L381 (7.4109, -3.0787) -> (7.4981, -3.0773)
  line L382 (7.4109, -3.0787) -> (7.3063, -3.0794)
  line L383 (7.3063, -3.0794) -> (7.4109, -3.0787)
  line L384 (7.3063, -3.0794) -> (7.1845, -3.0801)
  line L385 (7.1845, -3.0801) -> (7.3063, -3.0794)
  line L386 (7.1845, -3.0801) -> (6.6921, -3.0801)
  line L387 (6.6921, -3.0801) -> (7.1845, -3.0801)
  line L388 (6.6921, -3.0801) -> (6.881, -2.1797)
  line L389 (6.881, -2.1797) -> (6.6921, -3.0801)
  line L390 (6.881, -2.1797) -> (7.7497, -2.1797)
  line L391 (7.7497, -2.1797) -> (6.881, -2.1797)
  line L392 (7.7497, -2.1797) -> (7.8031, -2.1804)
  line L393 (7.8031, -2.1804) -> (7.7497, -2.1797)
  line L394 (7.7497, -2.1797) -> (7.8031, -2.1804)
  line L395 (7.8031, -2.1804) -> (7.9026, -2.1854)
  line L396 (7.9026, -2.1854) -> (7.9819, -2.1955)
  line L397 (7.9819, -2.1955) -> (8.041, -2.2107)
  line L398 (8.041, -2.2107) -> (8.0561, -2.2172)
  line L399 (8.0561, -2.2172) -> (8.1246, -2.2604)
  line L400 (8.1246, -2.2604) -> (8.1787, -2.3268)
  line L401 (8.1787, -2.3268) -> (8.1989, -2.365)
  line L402 (8.1989, -2.365) -> (8.2234, -2.4435)
  line L403 (8.2234, -2.4435) -> (8.2313, -2.5308)
  line L404 (8.2313, -2.5308) -> (8.2313, -2.5495)
  line L405 (8.2313, -2.5495) -> (8.2212, -2.6332)
  line L406 (8.2212, -2.6332) -> (8.1982, -2.7125)
  line L407 (8.1982, -2.7125) -> (8.1607, -2.7889)
  line L408 (8.1607, -2.7889) -> (8.1463, -2.812)
  line L409 (8.1463, -2.812) -> (8.0951, -2.8768)
  line L410 (8.0951, -2.8768) -> (8.0331, -2.9331)
  line L411 (8.0331, -2.9331) -> (7.961, -2.9799)
  line L412 (7.961, -2.9799) -> (7.9552, -2.9828)
  line L413 (7.9552, -2.9828) -> (7.8867, -3.0138)
  line L414 (7.8867, -3.0138) -> (7.8103, -3.0391)
  line L415 (7.8103, -3.0391) -> (7.7245, -3.0578)
  line L416 (7.7245, -3.0578) -> (7.6301, -3.0708)
  line L417 (7.6301, -3.0708) -> (7.62, -3.0715)
  line L418 (7.62, -3.0715) -> (7.5673, -3.0744)
  line L419 (7.5673, -3.0744) -> (7.4981, -3.0773)
  line L420 (7.4981, -3.0773) -> (7.4109, -3.0787)
  line L421 (7.4109, -3.0787) -> (7.3063, -3.0794)
  line L422 (7.3063, -3.0794) -> (7.1845, -3.0801)
  line L423 (7.1845, -3.0801) -> (6.6921, -3.0801)
  line L424 (6.6921, -3.0801) -> (6.881, -2.1797)
  line L425 (6.881, -2.1797) -> (7.7497, -2.1797)
  line L426 (7.8031, -2.1804) -> (7.7497, -2.1797)
  line L427 (7.7497, -2.1797) -> (6.881, -2.1797)
  line L428 (6.881, -2.1797) -> (6.6921, -3.0801)
  line L429 (6.6921, -3.0801) -> (7.1845, -3.0801)
  line L430 (7.1845, -3.0801) -> (7.3063, -3.0794)
  line L431 (7.3063, -3.0794) -> (7.4109, -3.0787)
  line L432 (7.4109, -3.0787) -> (7.4981, -3.0773)
  line L433 (7.4981, -3.0773) -> (7.5673, -3.0744)
  line L434 (7.5673, -3.0744) -> (7.62, -3.0715)
  line L435 (7.62, -3.0715) -> (7.6301, -3.0708)
  line L436 (7.6301, -3.0708) -> (7.7245, -3.0578)
  line L437 (7.7245, -3.0578) -> (7.8103, -3.0391)
  line L438 (7.8103, -3.0391) -> (7.8867, -3.0138)
  line L439 (7.8867, -3.0138) -> (7.9552, -2.9828)
  line L440 (7.9552, -2.9828) -> (7.961, -2.9799)
  line L441 (7.961, -2.9799) -> (8.0331, -2.9331)
  line L442 (8.0331, -2.9331) -> (8.0951, -2.8768)
  line L443 (8.0951, -2.8768) -> (8.1463, -2.812)
  line L444 (8.1463, -2.812) -> (8.1607, -2.7889)
  line L445 (8.1607, -2.7889) -> (8.1982, -2.7125)
  line L446 (8.1982, -2.7125) -> (8.2212, -2.6332)
  line L447 (8.2212, -2.6332) -> (8.2313, -2.5495)
  line L448 (8.2313, -2.5495) -> (8.2313, -2.5308)
  line L449 (8.2313, -2.5308) -> (8.2234, -2.4435)
  line L450 (8.2234, -2.4435) -> (8.1989, -2.365)
  line L451 (8.1989, -2.365) -> (8.1787, -2.3268)
  line L452 (8.1787, -2.3268) -> (8.1246, -2.2604)
  line L453 (8.1246, -2.2604) -> (8.0561, -2.2172)
  line L454 (8.0561, -2.2172) -> (8.041, -2.2107)
  line L455 (8.041, -2.2107) -> (7.9819, -2.1955)
  line L456 (7.9819, -2.1955) -> (7.9026, -2.1854)
  line L457 (7.9026, -2.1854) -> (7.8031, -2.1804)
  line L458 (0.7957, 9.0333) -> (1.2479, 10.4251)
  line L459 (0.7957, 9.0333) -> (1.2479, 10.4251)
  line L460 (-1.0969, 9.0333) -> (0.7957, 9.0333)
  line L461 (-1.0969, 9.0333) -> (0.7957, 9.0333)
  line L462 (-3.1926, 2.5833) -> (-1.0969, 9.0333)
  line L463 (-3.1926, 2.5833) -> (-1.0969, 9.0333)
  line L464 (-1.3, 2.5833) -> (-3.1926, 2.5833)
  line L465 (-1.3, 2.5833) -> (-3.1926, 2.5833)
  line L466 (-1.8363, 0.9327) -> (-1.3, 2.5833)
  line L467 (-1.8363, 0.9327) -> (-1.3, 2.5833)
  arc A1 (1.2479, 10.4251) -> (-1.8363, 0.9327) centre (0, 5.5833) ccw
  line L468 (-1.8363, 0.9327) -> (-1.3, 2.5833)
  line L469 (-1.3, 2.5833) -> (-3.1926, 2.5833)
  line L470 (-3.1926, 2.5833) -> (-1.0969, 9.0333)
  line L471 (-1.0969, 9.0333) -> (0.7957, 9.0333)
  line L472 (0.7957, 9.0333) -> (1.2479, 10.4251)
  arc A2 (1.2479, 10.4251) -> (-1.8363, 0.9327) centre (0, 5.5833) ccw
  line L473 (0.7957, 9.0333) -> (1.2479, 10.4251)
  line L474 (-1.0969, 9.0333) -> (0.7957, 9.0333)
  line L475 (-3.1926, 2.5833) -> (-1.0969, 9.0333)
  line L476 (-1.3, 2.5833) -> (-3.1926, 2.5833)
  line L477 (-1.8363, 0.9327) -> (-1.3, 2.5833)
  line L478 (2.1463, 10.0992) -> (1.8, 9.0333)
  line L479 (2.1463, 10.0992) -> (1.8, 9.0333)
  line L480 (-0.34, 2.5833) -> (-0.9596, 0.6763)
  line L481 (-0.34, 2.5833) -> (-0.9596, 0.6763)
  line L482 (1.76, 2.5833) -> (-0.34, 2.5833)
  line L483 (1.76, 2.5833) -> (-0.34, 2.5833)
  arc A3 (1.76, 2.5833) -> (2.5364, 6.4182) centre (1.4, 4.6522) ccw
  line L484 (1.76, 2.5833) -> (-0.34, 2.5833)
  line L485 (-0.34, 2.5833) -> (-0.9596, 0.6763)
  arc A4 (-0.9596, 0.6763) -> (2.1463, 10.0992) centre (0, 5.5833) ccw
  line L486 (2.1463, 10.0992) -> (1.8, 9.0333)
  arc A5 (2.5364, 6.4182) -> (1.8, 9.0333) centre (1.5559, 7.5533) ccw
  arc A6 (1.76, 2.5833) -> (2.5364, 6.4182) centre (1.4, 4.6522) ccw
  arc A7 (2.5364, 6.4182) -> (1.8, 9.0333) centre (1.5559, 7.5533) ccw
  line L487 (2.1463, 10.0992) -> (1.8, 9.0333)
  arc A8 (-0.9596, 0.6763) -> (2.1463, 10.0992) centre (0, 5.5833) ccw
  line L488 (-0.34, 2.5833) -> (-0.9596, 0.6763)
  line L489 (1.76, 2.5833) -> (-0.34, 2.5833)
  line L490 (-0.34, 2.5833) -> (1.8, 9.0333)
  line L491 (-0.34, 2.5833) -> (1.8, 9.0333)
  line L492 (-1.3, 2.5833) -> (-0.34, 2.5833)
  line L493 (-1.3, 2.5833) -> (-0.34, 2.5833)
  line L494 (0.7957, 9.0333) -> (-1.3, 2.5833)
  line L495 (0.7957, 9.0333) -> (-1.3, 2.5833)
  line L496 (1.8, 9.0333) -> (0.7957, 9.0333)
  line L497 (1.8, 9.0333) -> (0.7957, 9.0333)
  line L498 (1.8, 9.0333) -> (0.7957, 9.0333)
  line L499 (0.7957, 9.0333) -> (-1.3, 2.5833)
  line L500 (-1.3, 2.5833) -> (-0.34, 2.5833)
  line L501 (-0.34, 2.5833) -> (1.8, 9.0333)
  line L502 (1.8, 9.0333) -> (0.7957, 9.0333)
  line L503 (-0.34, 2.5833) -> (1.8, 9.0333)
  line L504 (-1.3, 2.5833) -> (-0.34, 2.5833)
  line L505 (0.7957, 9.0333) -> (-1.3, 2.5833)
  line L506 (-14.3666, -1.5833) -> (-16.4058, -1.5833)
  line L507 (-16.4058, -1.5833) -> (-14.3666, -1.5833)
  arc A9 (-14.2731, -2.9167) -> (-14.3666, -1.5833) centre (-14.3962, -2.2554) ccw
  arc A10 (-14.2731, -2.9167) -> (-14.3666, -1.5833) centre (-14.3962, -2.2554) ccw
  arc A11 (-13.78, -3.5707) -> (-14.2731, -2.9167) centre (-14.4006, -3.5257) ccw
  arc A12 (-13.78, -3.5707) -> (-14.2731, -2.9167) centre (-14.4006, -3.5257) ccw
  arc A13 (-14.9696, -4.5833) -> (-13.78, -3.5707) centre (-14.9493, -3.4022) ccw
  arc A14 (-14.9696, -4.5833) -> (-13.78, -3.5707) centre (-14.9493, -3.4022) ccw
  line L508 (-16.9348, -4.5833) -> (-14.9696, -4.5833)
  line L509 (-14.9696, -4.5833) -> (-16.9348, -4.5833)
  line L510 (-16.4058, -1.5833) -> (-16.9348, -4.5833)
  line L511 (-16.9348, -4.5833) -> (-16.4058, -1.5833)
  line L512 (-13.2133, -3.1067) -> (-13.2869, -3.5243)
  line L513 (-13.2869, -3.5243) -> (-13.2133, -3.1067)
  ellipse E0 centre (-11.6332, -3.3214) end of major axis (-13.2367, -3.3214) minor radius 1.2619 (-11.6332, -2.0595) -> (-13.2133, -3.1067) ccw
  ellipse E1 centre (-11.6332, -3.3214) end of major axis (-13.2367, -3.3214) minor radius 1.2619 (-11.6332, -2.0595) -> (-13.2133, -3.1067) ccw
  line L514 (-11.3012, -2.0595) -> (-11.6332, -2.0595)
  line L515 (-11.6332, -2.0595) -> (-11.3012, -2.0595)
  arc A15 (-10.4058, -3.1185) -> (-11.3012, -2.0595) centre (-11.3012, -2.9675) ccw
  arc A16 (-10.4058, -3.1185) -> (-11.3012, -2.0595) centre (-11.3012, -2.9675) ccw
  line L516 (-10.4532, -3.3962) -> (-10.4058, -3.1185)
  line L517 (-10.4058, -3.1185) -> (-10.4532, -3.3962)